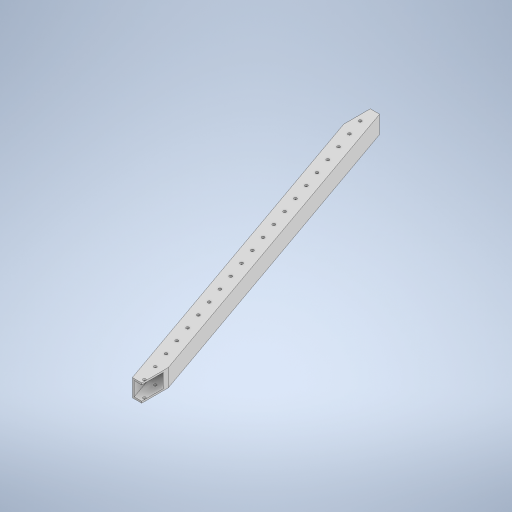
# Autodesk Inventor part: 1 x 1 x 0.100 Pre-drilled stock ( angled)
Saved by Autodesk Inventor 2023 (Build 270158030, 158C)
## iProperties
Created: 2022-07-22
Part Number: 1 x 1 x 0.100 Pre-drilled stock ( angled)
Material: Generic
Document SubType Name: Modeling
Designer: kt1040502
Density: 1 g/cm^3
Appearance: Default
Author: kt1040502
Autodesk Inventor part; units mm, degrees
ref_plane "YZ Plane" through (0, 0, 0) normal (1, 0, 0) x (0, 1, 0)
ref_plane "XZ Plane" through (0, 0, 0) normal (0, 1, 0) x (-1, 0, 0)
ref_plane "XY Plane" through (0, 0, 0) normal (0, 0, 1) x (1, 0, 0)
sketch "Sketch1" plane through (0, 0, 0) normal (0, 1, 0) x (-1, 0, 0)
  line L0 (0, 0) -> (177.8, 0)
  line L1 (177.8, 0) -> (177.8, -508)
  line L2 (177.8, -508) -> (0, -508)
  line L3 (0, -508) -> (0, 0)
  line L4 (11.987, 4.1955) -> (189.787, -503.8045)
  line L5 (-11.987, -4.1955) -> (165.813, -512.1955)
  line L6 (0, -38.444) -> (164.3446, -508)
  line L7 (177.8, -469.556) -> (13.4554, 0)
  line L8 (-11.987, -4.1955) -> (11.987, 4.1955)
  line L9 (189.787, -503.8045) -> (165.813, -512.1955)
  line L10 (0, 0) -> (2.0977, -5.9935)
  circle A0 centre (2.0977, -5.9935) radius 2.032
  line L11 (2.0977, -5.9935) -> (10.4886, -29.9675)
  circle A1 centre (10.4886, -29.9675) radius 2.032
  line L12 (10.4886, -29.9675) -> (18.8795, -53.9415)
  circle A2 centre (18.8795, -53.9415) radius 2.032
  line L13 (18.8795, -53.9415) -> (27.2704, -77.9155)
  circle A3 centre (27.2704, -77.9155) radius 2.032
  line L14 (27.2704, -77.9155) -> (35.6613, -101.8895)
  circle A4 centre (35.6613, -101.8895) radius 2.032
  line L15 (35.6613, -101.8895) -> (177.8, -508)
  line L16 (27.2704, -77.9155) -> (35.6613, -101.8895)
  circle A5 centre (35.6613, -101.8895) radius 2.032
  line L17 (35.6613, -101.8895) -> (44.0522, -125.8635)
  circle A6 centre (44.0522, -125.8635) radius 2.032
  line L18 (35.6613, -101.8895) -> (44.0522, -125.8635)
  circle A7 centre (44.0522, -125.8635) radius 2.032
  line L19 (44.0522, -125.8635) -> (52.4431, -149.8375)
  circle A8 centre (52.4431, -149.8375) radius 2.032
  line L20 (44.0522, -125.8635) -> (52.4431, -149.8375)
  circle A9 centre (52.4431, -149.8375) radius 2.032
  line L21 (52.4431, -149.8375) -> (60.834, -173.8115)
  circle A10 centre (60.834, -173.8115) radius 2.032
  line L22 (52.4431, -149.8375) -> (60.834, -173.8115)
  circle A11 centre (60.834, -173.8115) radius 2.032
  line L23 (60.834, -173.8115) -> (69.2249, -197.7855)
  circle A12 centre (69.2249, -197.7855) radius 2.032
  line L24 (60.834, -173.8115) -> (69.2249, -197.7855)
  circle A13 centre (69.2249, -197.7855) radius 2.032
  line L25 (69.2249, -197.7855) -> (77.6158, -221.7595)
  circle A14 centre (77.6158, -221.7595) radius 2.032
  line L26 (69.2249, -197.7855) -> (77.6158, -221.7595)
  circle A15 centre (77.6158, -221.7595) radius 2.032
  line L27 (77.6158, -221.7595) -> (86.0067, -245.7335)
  circle A16 centre (86.0067, -245.7335) radius 2.032
  line L28 (77.6158, -221.7595) -> (86.0067, -245.7335)
  circle A17 centre (86.0067, -245.7335) radius 2.032
  line L29 (86.0067, -245.7335) -> (94.3976, -269.7075)
  circle A18 centre (94.3976, -269.7075) radius 2.032
  line L30 (86.0067, -245.7335) -> (94.3976, -269.7075)
  circle A19 centre (94.3976, -269.7075) radius 2.032
  line L31 (94.3976, -269.7075) -> (102.7885, -293.6815)
  circle A20 centre (102.7885, -293.6815) radius 2.032
  line L32 (94.3976, -269.7075) -> (102.7885, -293.6815)
  circle A21 centre (102.7885, -293.6815) radius 2.032
  line L33 (102.7885, -293.6815) -> (111.1794, -317.6555)
  circle A22 centre (111.1794, -317.6555) radius 2.032
  line L34 (102.7885, -293.6815) -> (111.1794, -317.6555)
  circle A23 centre (111.1794, -317.6555) radius 2.032
  line L35 (111.1794, -317.6555) -> (119.5703, -341.6295)
  circle A24 centre (119.5703, -341.6295) radius 2.032
  line L36 (111.1794, -317.6555) -> (119.5703, -341.6295)
  circle A25 centre (119.5703, -341.6295) radius 2.032
  line L37 (119.5703, -341.6295) -> (127.9612, -365.6035)
  circle A26 centre (127.9612, -365.6035) radius 2.032
  line L38 (119.5703, -341.6295) -> (127.9612, -365.6035)
  circle A27 centre (127.9612, -365.6035) radius 2.032
  line L39 (127.9612, -365.6035) -> (136.3521, -389.5775)
  circle A28 centre (136.3521, -389.5775) radius 2.032
  line L40 (127.9612, -365.6035) -> (136.3521, -389.5775)
  circle A29 centre (136.3521, -389.5775) radius 2.032
  line L41 (136.3521, -389.5775) -> (144.743, -413.5515)
  circle A30 centre (144.743, -413.5515) radius 2.032
  line L42 (136.3521, -389.5775) -> (144.743, -413.5515)
  circle A31 centre (144.743, -413.5515) radius 2.032
  line L43 (144.743, -413.5515) -> (153.1339, -437.5255)
  circle A32 centre (153.1339, -437.5255) radius 2.032
  line L44 (144.743, -413.5515) -> (153.1339, -437.5255)
  circle A33 centre (153.1339, -437.5255) radius 2.032
  line L45 (153.1339, -437.5255) -> (161.5248, -461.4995)
  circle A34 centre (161.5248, -461.4995) radius 2.032
  line L46 (153.1339, -437.5255) -> (161.5248, -461.4995)
  circle A35 centre (161.5248, -461.4995) radius 2.032
  line L47 (161.5248, -461.4995) -> (169.9157, -485.4735)
  circle A36 centre (169.9157, -485.4735) radius 2.032
  dimension "d0" = 177.8
  dimension "d1" = 508
  dimension "d19" = 25.4
  constraints: 96 end point, 37 centre point, 37 coincident, 9 point on line, 3 parallel, 1 horizontal, 1 perpendicular, 145 other
  measures "d0" distance of L1.end L2.end
  measures "d1" distance of L0.end L1.end
  measures "d19" distance of L13.start L16.start
extrude "Extrusion1" add sketch "Sketch1" against normal blind 25.4 contours L8 L4 L0 | L10 A0 L11 A1 L12 A2 L13 A3 L14 A4 L15 A6 A8 A10 A12 A14 A16 A18 A20 A22 A24 A26 A28 A30 A32 A34 A36 L2 L5 L3 | L0 L4 L1 L15 A36 A34 A32 A30 A28 A26 A24 A22 A20 A18 A16 A14 A12 A10 A8 A6 A4 L14 A3 L13 A2 L12 A1 L11 A0 L10
sketch "Sketch3" plane through (-11.987, -25.4, 4.1955) normal (0.3304, 0, 0.9439) x (0.9439, 0, -0.3304)
  line L0 (0, 25.4) -> (0, 0) projected
  line L1 (25.4, 25.4) -> (25.4, 0) projected
  line L2 (0, 25.4) -> (25.4, 25.4)
  line L3 (25.4, 25.4) -> (25.4, 0)
  line L4 (25.4, 0) -> (0, 0)
  line L5 (0, 0) -> (0, 25.4)
  line L6 (0, 25.4) -> (2.54, 25.4)
  line L7 (0, 25.4) -> (12.7, 25.4) projected
  line L8 (25.4, 0) -> (22.86, 0)
  line L9 (25.4, 0) -> (12.7, 0) projected
  line L10 (2.54, 25.4) -> (22.86, 25.4)
  line L11 (22.86, 0) -> (2.54, 0)
  line L12 (2.54, 25.4) -> (2.54, 22.86)
  line L13 (22.86, 0) -> (22.86, 2.54)
  line L14 (2.54, 22.86) -> (22.86, 22.86)
  line L15 (22.86, 22.86) -> (22.86, 2.54)
  line L16 (22.86, 2.54) -> (2.54, 2.54)
  line L17 (2.54, 2.54) -> (2.54, 22.86)
  dimension "d23" = 25.4
  dimension "d24" = 25.4
  dimension "d25" = 2.54
  dimension "d26" = 2.54
  dimension "d27" = 2.54
  dimension "d28" = 2.54
  constraints: 28 end point, 5 parallel, 4 perpendicular, 3 horizontal, 2 point on line
  measures "d23" distance of L1.end L4.end
  measures "d24" distance of L2.end L1.end
  measures "d25" distance of L0.start L6.end
  measures "d26" distance of L1.end L8.end
  measures "d27" distance of L6.end L12.end
  measures "d28" distance of L8.end L13.end
extrude "Extrusion2" cut sketch "Sketch3" against normal blind 556.26 contours L14 L15 L16 L17
extrude "Extrusion3" cut sketch "Sketch1" against normal blind 25.4 contours L8 L4 L0
body "Solid1"
